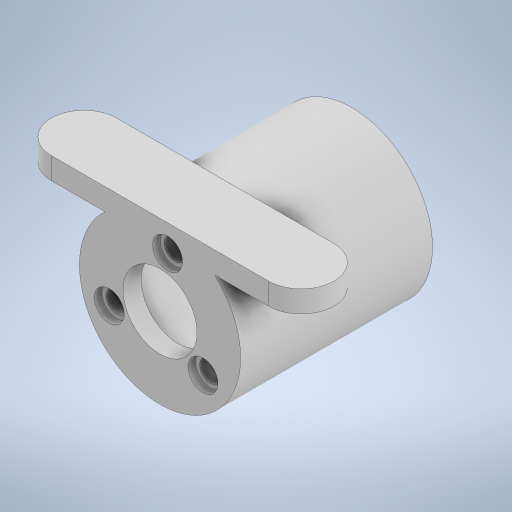
# Autodesk Inventor part: v5motormount
Saved by Autodesk Inventor 2024.2 (Build 282272000, 272)
## iProperties
Created: 2024-04-07
Part Number: v5motormount
Material: Generic
Document SubType Name: Modeling
Designer: Eric
Density: 1 g/cm^3
Appearance: Default
Author: Eric
Autodesk Inventor part; units mm, degrees
ref_plane "YZ Plane" through (0, 0, 0) normal (1, 0, 0) x (0, 1, 0)
ref_plane "XY Plane" through (0, 0, 0) normal (0, 0, 1) x (1, 0, 0)
sketch "Sketch1" plane through (0, 0, 0) normal (0, 0, 1) x (1, 0, 0)
  circle A0 centre (0, 0) radius 5.1
  circle A1 centre (1.0508, 7.4765) radius 1.45
  circle A2 centre (-7.0002, -2.8283) radius 1.45
  circle A3 centre (5.9495, -4.6482) radius 1.45
  line L0 (0, 0) -> (0, 9.6313) construction
  line L1 (1.0508, 7.4765) -> (0, 0) construction
  circle A4 centre (0, 0) radius 11.125
  dimension "d0" = 10.2
  dimension "d1" = 2.9
  dimension "d2" = 7.55
  dimension "d5" = 360
  dimension "d7" = 8
  dimension "d8" = 22.25
  constraints: 5 centre point, 4 end point, 2 coincident, 1 vertical, 7 other
  measures "d0" diameter of A0
  measures "d1" diameter of A1
  measures "d2" distance of point (0, 0) L1.start
  measures "d7" angle of L0 L1
  measures "d8" diameter of A4
extrude "Extrusion1" add sketch "Sketch1" along normal blind 1.5 contours A1 | A2 | A3 | A4
sketch "Sketch2" plane through (0, 0, 1.5) normal (0, 0, 1) x (1, 0, 0)
  circle A0 centre (0, 0) radius 11.125 projected
  circle A1 centre (0, 0) radius 5.1 projected
  circle A2 centre (1.0508, 7.4765) radius 1.45 projected
  circle A3 centre (-7.0002, -2.8283) radius 1.45 projected
  circle A4 centre (5.9495, -4.6482) radius 1.45 projected
  circle A5 centre (-7.0002, -2.8283) radius 2.05
  circle A6 centre (1.0508, 7.4765) radius 2.05
  circle A7 centre (5.9495, -4.6482) radius 2.05
  dimension "d11" = 4.1
  constraints: 3 centre point, 3 coincident, 2 equal radius
  measures "d11" diameter of A5
extrude "Extrusion2" add sketch "Sketch2" along normal blind 1 contours A0 | A2 | A3 | A4 | A5 | A6 | A7
sketch "Sketch3" plane through (0, 0, 0) normal (0, 0, -1) x (-1, 0, 0)
  circle A0 centre (0, 0) radius 11.125 projected
  circle A1 centre (0, 0) radius 10.125
  dimension "d14" = 20.25
  constraints: 1 centre point, 1 coincident
  measures "d14" diameter of A1
extrude "Extrusion3" add sketch "Sketch3" along normal blind 24
ref_plane "Work Plane1" through (0, 11.125, 0) normal (0, 1, 0) x (-1, 0, 0)
sketch "Sketch4" plane through (0, 11.125, 0) normal (0, 1, 0) x (-1, 0, 0)
  circle A0 centre (15, -2) radius 4.5
  circle A1 centre (-15, -2) radius 4.5
  line L0 (15, 2.5) -> (-15, 2.5)
  line L1 (15, -6.5) -> (-15, -6.5)
  line L2 (11.125, 2.5) -> (-11.125, 2.5) projected
  point P0 (0, 0)
  point P1 (0, 2.5)
  dimension "d18" = 9
  dimension "d19" = 30
  dimension "d20" = 15
  constraints: 4 end point, 4 point on circle, 2 centre point, 2 tangent, 1 collinear, 1 equal radius, 1 horizontal, 1 midpoint
  measures "d18" diameter of A0
  measures "d19" distance of A1.centre A0.centre
  measures "d20" horizontal distance of point (0, 2.5) A0.centre
extrude "Extrusion4" add sketch "Sketch4" against normal blind 3
sketch "Sketch5" plane through (0, 0, -24) normal (0, 0, -1) x (-1, 0, 0)
  circle A0 centre (0, 0) radius 10.125 projected
extrude "Extrusion5" cut sketch "Sketch5" against normal up to surface (24 mm away)
sketch "Sketch6" plane through (0, 0, 2.5) normal (0, 0, 1) x (1, 0, 0)
  circle A0 centre (1.0508, 7.4765) radius 1.45 projected
  circle A1 centre (5.9495, -4.6482) radius 1.45 projected
  circle A2 centre (-7.0002, -2.8283) radius 1.45 projected
  point P0 (0, 0)
hole "Hole1" at (-7.0002, -2.8283, 2.5) at (1.0508, 7.4765, 2.5) at (5.9495, -4.6482, 2.5) direction (0, 0, -1) diameter 2.9 end through all counterbore diameter 4.1 counterbore depth 1
body "Solid1"
